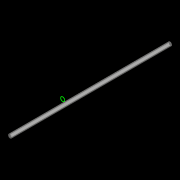
# Autodesk Inventor part: Diffusion Foam
Saved by Autodesk Inventor 2022.1 (Build 261234000, 234)
## iProperties
Created: 2022-01-31
Part Number: Diffusion Foam
Material: Polycarbonate, Smoke
Document SubType Name: Modeling
Designer: Michael Lacey
Mass: 279.037 g
Surface Area: 981.735 cm^2
Volume: 232.531 cm^3
Density: 1.2 g/cm^3
Appearance: Polycarbonate - Smoked
Author: Michael Lacey
Autodesk Inventor part; units mm, degrees
ref_plane "YZ Plane" through (0, 0, 0) normal (1, 0, 0) x (0, 1, 0)
ref_plane "XZ Plane" through (0, 0, 0) normal (0, 1, 0) x (-1, 0, 0)
ref_plane "XY Plane" through (0, 0, 0) normal (0, 0, 1) x (1, 0, 0)
sketch "Sketch1" plane through (0, 0, 0) normal (0, 0, 1) x (1, 0, 0)
  circle A0 centre (0, 0) radius 11.1125
  circle A1 centre (0, 0) radius 6.35
  dimension "d0" = 22.225
  dimension "d1" = 12.7
  constraints: 2 centre point, 2 coincident
  measures "d0" diameter of A0
  measures "d1" diameter of A1
extrude "Extrusion1" add sketch "Sketch1" against normal blind 890
body "Solid1"
